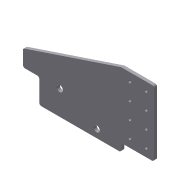
# Autodesk Inventor part: Frame_BottomRollerPlate
Saved by Autodesk Inventor 2012 (Build 160160000, 160)
## iProperties
Created: 2012-01-09
Part Number: Frame_BottomRollerPlate
Material: Aluminum-6061
Document SubType Name: Modeling
Designer: JesseK
Mass: 225.209 g
Surface Area: 385.27 cm^2
Volume: 83.1028 cm^3
Density: 2.71 g/cm^3
Author: JesseK
Autodesk Inventor part; units mm, degrees
ref_plane "YZ Plane" through (0, 0, 0) normal (1, 0, 0) x (0, 1, 0)
ref_plane "XZ Plane" through (0, 0, 0) normal (0, 1, 0) x (-1, 0, 0)
ref_plane "XY Plane" through (0, 0, 0) normal (0, 0, 1) x (1, 0, 0)
sketch "Sketch1" plane through (0, 0, 0) normal (0, 0, 1) x (1, 0, 0)
  line L0 (0, 0) -> (203.2, 0)
  line L1 (203.2, 0) -> (203.2, 127)
  line L2 (203.2, 127) -> (0, 127)
  line L3 (0, 127) -> (0, 0)
  dimension "d0" = 203.2
  dimension "d1" = 127
  constraints: 8 end point, 2 parallel, 1 horizontal, 1 perpendicular
  measures "d0" distance of L0.start L0.end
  measures "d1" distance of L2.end L0.start
extrude "Extrusion1" add sketch "Sketch1" along normal blind 4.7625
sketch "Sketch2" plane through (0, 0, 4.7625) normal (0, 0, 1) x (1, 0, 0)
  line L0 (203.2, 127) -> (203.2, 0) projected
  line L1 (0, 127) -> (203.2, 127) projected
  line L2 (190.5, 127) -> (190.5, 101.6) construction
  circle A0 centre (190.5, 101.6) radius 2.3813
  dimension "d4" = 4.7625
  dimension "d5" = 25.4
  dimension "d6" = 12.7
  constraints: 2 end point, 1 centre point, 1 coincident, 1 perpendicular, 1 point on line
  measures "d4" diameter of A0
  measures "d5" distance of L2.start L2.end
  measures "d6" distance from line of L0 L2.end
extrude "Extrusion2" cut sketch "Sketch2" against normal up to next
pattern_linear "Rectangular Pattern1" count 4 spacing 25.4 along (0, -1, 0) count 2 spacing 25.4 along (-1, 0, 0) of "Extrusion2"
sketch "Sketch3" plane through (0, 0, 4.7625) normal (0, 0, 1) x (1, 0, 0)
  line L0 (203.2, 0) -> (0, 0) projected
  line L1 (203.2, 127) -> (203.2, 0) projected
  circle A0 centre (114.3, 12.7) radius 4.7625
  circle A1 centre (57.15, 38.1) radius 4.7625
  dimension "d15" = 9.525
  dimension "d16" = 88.9
  dimension "d17" = 12.7
  dimension "d18" = 57.15
  dimension "d19" = 25.4
  constraints: 2 centre point, 1 equal radius
  measures "d15" diameter of A0
  measures "d16" distance from line of L1 A0.centre
  measures "d17" distance from line of L0 A0.centre
  measures "d18" horizontal distance of A0.centre A1.centre
  measures "d19" vertical distance of A0.centre A1.centre
extrude "Extrusion3" cut sketch "Sketch3" against normal up to next
sketch "Sketch4" plane through (0, 0, 4.7625) normal (0, 0, 1) x (1, 0, 0)
  line L0 (0, 0) -> (0, 127) projected
  line L1 (0, 0) -> (25.4, 0)
  line L2 (25.4, 0) -> (25.4, 38.1)
  line L3 (25.4, 38.1) -> (0, 38.1)
  line L4 (0, 38.1) -> (0, 0)
  line L5 (203.2, 127) -> (0, 127)
  line L6 (0, 127) -> (0, 114.3)
  line L7 (0, 114.3) -> (203.2, 114.3)
  line L8 (203.2, 114.3) -> (203.2, 127)
  line L9 (203.2, 0) -> (152.4, 0)
  line L10 (152.4, 0) -> (152.4, 12.7)
  line L11 (152.4, 12.7) -> (203.2, 12.7)
  line L12 (203.2, 12.7) -> (203.2, 0)
  dimension "d22" = 38.1
  dimension "d23" = 25.4
  dimension "d24" = 50.8
  dimension "d25" = 12.7
  dimension "d26" = 12.7
  constraints: 24 end point, 6 parallel, 3 horizontal, 3 perpendicular, 1 point on line
  measures "d22" distance of L1.end L2.end
  measures "d23" distance of L2.end L3.end
  measures "d24" distance of L10.end L11.end
  measures "d25" distance of L9.end L10.end
  measures "d26" distance of L6.end L0.end
extrude "Extrusion4" cut sketch "Sketch4" against normal up to next
sketch "Sketch5" plane through (0, 0, 4.7625) normal (0, 0, 1) x (1, 0, 0)
  line L0 (203.2, 114.3) -> (0, 114.3) projected
  line L1 (0, 38.1) -> (0, 114.3) projected
  line L2 (0, 114.3) -> (0, 63.5)
  line L3 (152.4, 114.3) -> (0, 63.5)
  line L4 (0, 114.3) -> (152.4, 114.3)
  point P0 (0, 0)
  dimension "d29" = 25.4
  dimension "d30" = 50.8
  constraints: 6 end point, 2 point on line, 1 collinear
  measures "d29" distance of L1.start L2.end
  measures "d30" distance of L0.start L3.start
extrude "Extrusion5" cut sketch "Sketch5" against normal up to next
fillet "Fillet1" radius 3.175 9 edges at (0, 63.5, 2.3813) (0, 38.1, 2.3813) (25.4, 0, 2.3813) (152.4, 114.3, 2.3813) (203.2, 114.3, 2.3813) (203.2, 12.7, 2.3813) (152.4, 12.7, 2.3813) (152.4, 0, 2.3813) (25.4, 38.1, 2.3813)
body "Solid1"
